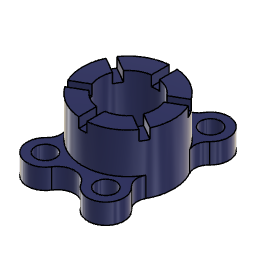
Design 1 v1 (Autodesk Fusion 360 design; units mm, degrees)
Autodesk Fusion 360 part; units mm, degrees
note: some values were not read from the file. Set by a fixed rule: which sketch regions a step uses.
sketch "Sketch1" plane through (0, 0, 0) normal (0, 0, 1) x (1, 0, 0)
  circle A0 centre (0, 0) radius 27.5
  circle A1 centre (0, 0) radius 45
  line L0 (0, 0) -> (0, 80) construction
  line L1 (0, 0) -> (70, 0) construction
  line L2 (0, 0) -> (-41.7412, 72.298) construction
  circle A2 centre (-30, 51.9615) radius 10
  circle A3 centre (30, 51.9615) radius 10
  arc A4 (-14.5714, 61.2329) -> (14.5714, 61.2329) centre (0, 69.9893) ccw
  arc A5 (-39.4278, 21.6899) -> (-42.203, 38.7295) centre (-51.6942, 28.4379) ccw
  arc A6 (42.203, 38.7295) -> (39.4278, 21.6899) centre (51.6942, 28.4379) ccw
  arc A7 (-14.5714, 61.2329) -> (-42.203, 38.7295) centre (-30, 51.9615) ccw
  arc A8 (42.203, 38.7295) -> (14.5714, 61.2329) centre (30, 51.9615) ccw
  arc A9 (-42.203, -38.7295) -> (-39.4278, -21.6899) centre (-51.6942, -28.4379) ccw
  arc A10 (-42.203, -38.7295) -> (-14.5714, -61.2329) centre (-30, -51.9615) ccw
  arc A11 (14.5714, -61.2329) -> (-14.5714, -61.2329) centre (0, -69.9893) ccw
  arc A12 (14.5714, -61.2329) -> (42.203, -38.7295) centre (30, -51.9615) ccw
  arc A13 (39.4278, -21.6899) -> (42.203, -38.7295) centre (51.6942, -28.4379) ccw
  circle A14 centre (30, -51.9615) radius 10
  circle A15 centre (-30, -51.9615) radius 10
  dimension "d1" = 55
  dimension "d2" = 90
  dimension "d3" = 30
  dimension "d4" = 20
  dimension "d5" = 36
  dimension "d6" = 60
  dimension "d7" = 17
  dimension "d8" = 14
  constraint coincident A0.centre A1.centre
  constraint concentric A0 A1
  constraint vertical L0
  constraint perpendicular L0 L1
  constraint coincident L2 A2.centre
  constraint concentric A2 A7
  constraint symmetric L0 A2 A3
  constraint symmetric L0 A7 A8
  constraint tangent A4 A8
  constraint tangent A1 A5
  constraint coincident A1 A5.start
  constraint tangent A4 A7
  constraint tangent A5 A7
  constraint symmetric L0 A5.end A6.start
  constraint symmetric L0 A5.start A6.end
  constraint symmetric L0 A5 A6
  constraint symmetric L1 A2 A15
  constraint symmetric L1 A3 A14
  constraint symmetric L1 A4.start A10.end
  constraint symmetric L1 A4.end A11.start
  constraint symmetric L1 A4 A11
  constraint symmetric L1 A5.end A9.start
  constraint symmetric L1 A5.start A9.end
  constraint symmetric L1 A5 A9
  constraint symmetric L1 A6.end A13.start
  constraint symmetric L1 A6.start A12.end
  constraint symmetric L1 A6 A13
  constraint symmetric L1 A7 A10
  constraint symmetric L1 A8 A12
  measures "d1" diameter of A0
  measures "d2" diameter of A1
  measures "d3" angle of L0 L2
  measures "d4" diameter of A2
  measures "d5" diameter of A7
  measures "d6" distance of A0.centre A2.centre
  measures "d7" radius of A4
  measures "d8" radius of A5
extrude "Extrude1" add sketch "Sketch1" along normal blind 20 contours A1 A4 A5 A6 A7 A8 | A1 A9 A10 A11 A12 A13 makes body 1 at (17.6653, 41.3877, 13.3333) makes body 2 at (-19.6089, -40.503, 6.6667)
extrude "Extrude2" add sketch "Sketch1" along normal blind 60 contours A1 bodies 1 2
sketch "Sketch2" plane through (0, 0, 60) normal (0, 0, 1) x (-1, 0, 0)
  circle A0 centre (0, 0) radius 27.5
  circle A1 centre (0, 0) radius 45
  line L0 (4, -22.5) -> (-4, -22.5)
  line L1 (-4, -22.5) -> (-4, -47.5)
  line L2 (-4, -47.5) -> (4, -47.5)
  line L3 (4, -47.5) -> (4, -22.5)
  line L4 (4, -22.5) -> (-4, -47.5) construction
  line L5 (-4, -22.5) -> (4, -47.5) construction
  point P0 (0, -35)
  dimension "d13" = 8
  dimension "d14" = 25
  constraint horizontal L0
  constraint perpendicular L0 L1
  constraint parallel L0 L2
  constraint parallel L1 L3
  constraint coincident L4 P0
  constraint coincident L5 P0
  measures "d13" distance of L1.end L2.end
  measures "d14" distance of L0.end L1.end
extrude "Extrude3" cut sketch "Sketch2" against normal blind 10 contours A0 A1 L1 L3 picked at (-3.1125, -33.1656) bodies 1
pattern_circular "C-Pattern1" count 6 over 360 about axis through (0, 0, 60) along (0, 0, 1) of "Extrude3"
